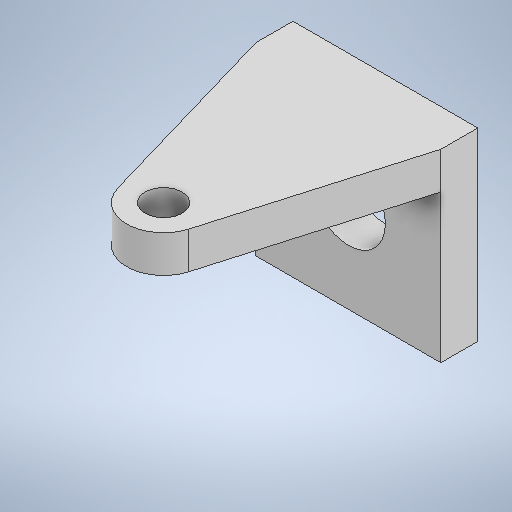
# Autodesk Inventor part: cad@35
Saved by Autodesk Inventor 2025.2 (Build 292293000, 293)
## iProperties
Created: 2025-03-24
Part Number: cad@35
Material: Generic
Document SubType Name: Modeling
Designer: spars
Density: 1 g/cm^3
Appearance: Default
Author: spars
Autodesk Inventor part; units mm, degrees
ref_plane "YZ Plane" through (0, 0, 0) normal (1, 0, 0) x (0, 1, 0)
ref_plane "XY Plane" through (0, 0, 0) normal (0, 0, 1) x (1, 0, 0)
sketch "Sketch1" plane through (0, 0, 0) normal (0, 0, 1) x (1, 0, 0)
  line L0 (-335.2657, 170.906) -> (-144.554, 170.906) construction
  line L1 (-144.554, 170.906) -> (-144.554, -100.0273) construction
  line L2 (-144.554, -100.0273) -> (-335.2657, -100.0273) construction
  line L3 (-335.2657, -100.0273) -> (-335.2657, 170.906) construction
  line L4 (-25, 25) -> (25, 25)
  line L5 (25, 25) -> (25, -25)
  line L6 (25, -25) -> (-25, -25)
  line L7 (-25, -25) -> (-25, 25)
  line L8 (-25, 25) -> (25, -25) construction
  line L9 (25, 25) -> (-25, -25) construction
  circle A0 centre (0, 0) radius 10
  dimension "d6" = 50
  dimension "d7" = 50
  dimension "d8" = 20
  constraints: 12 end point, 2 midpoint, 2 parallel, 1 centre point, 1 coincident, 1 horizontal, 1 perpendicular, 2 other
  measures "d6" distance of L5.end L6.end
  measures "d7" distance of L4.end L5.end
  measures "d8" diameter of A0
extrude "Extrusion1" add sketch "Sketch1" along normal blind 10
ref_plane "Work Plane1" through (0, 25, 0) normal (0, 1, 0) x (-1, 0, 0)
sketch "Sketch2" plane through (-25, 25, 0) normal (0, 1, 0) x (1, 0, 0)
  arc A0 (15.4, -62.8) -> (34.6, -62.8) centre (25, -60) ccw
  circle A1 centre (25, -60) radius 5
  line L0 (50, -10) -> (0, -10) projected
  line L1 (50, -10) -> (34.6, -62.8)
  line L2 (0, -10) -> (15.4, -62.8)
  line L3 (0, -10) -> (50, -10) projected
  line L4 (50, -10) -> (0, -10)
  line L5 (0, -10) -> (50, -10)
  point P0 (25, 0)
  dimension "d13" = 20
  dimension "d14" = 10
  dimension "d15" = 50
  constraints: 8 end point, 2 centre point, 2 collinear, 2 point on circle, 2 tangent, 1 coincident
  measures "d13" diameter of A0
  measures "d14" diameter of A1
  measures "d15" distance from line of L0 A0.centre
extrude "Extrusion2" add sketch "Sketch2" against normal blind 10
body "Solid1"
